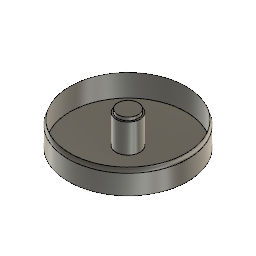
pot v3 (Autodesk Fusion 360 archive; units mm, degrees)
design "socle"
Autodesk Fusion 360 part; units mm, degrees
cylinder "CylindrePrimitive1" add diameter 75 height 15 placed x (1, 0, 0) y (0, 1, 0) z (0, 0, 1) at (0, 0, 0)
shell "Coque1" thickness 1 removed faces 1 at (9.3028, 10.3652, 15)
fillet "Congé1" radius 4 1 edges at (-34.9623, -13.5606, 15)
cylinder "CylindrePrimitive2" add diameter 15 height 20 placed x (1, 0, 0) y (0, 1, 0) z (0, 0, 1) at (0, 0, 1)
extrude "Extrusion1" cut 1 faces at (1.9158, 2.8099, 21) along direction (0, 0, -1) blind 2 thin wall 1 inside

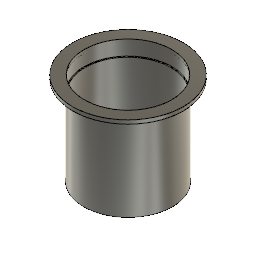
design "coffrage"
Autodesk Fusion 360 part; units mm, degrees
cylinder "CylindrePrimitive1" add diameter 60 height 60 placed x (1, 0, 0) y (0, 1, 0) z (0, 0, 1) at (0, 0, 0)
shell "Coque1" thickness 1 removed faces 1 at (7.6631, 11.2397, 60)
cylinder "CylindrePrimitive2" add diameter 75 height 2.5 placed x (1, 0, 0) y (0, 1, 0) z (0, 0, 1) at (0, 0, 60)
hole "Perçage1" at (0, 0, 62.5) direction (0, 0, -1) diameter 59 depth 10 tip angle 118
